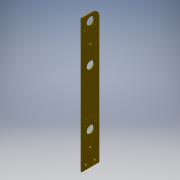
# Autodesk Inventor part: Back Plate
Saved by Autodesk Inventor 2017 (Build 210142000, 142)
## iProperties
Created: 2017-01-13
Part Number: Back Plate
Material: Generic
Document SubType Name: Modeling
Designer: Ben
Density: 1 g/cm^3
Appearance: Gold
Author: Ben
Autodesk Inventor part; units mm, degrees
ref_plane "YZ Plane" through (0, 0, 0) normal (1, 0, 0) x (0, 1, 0)
ref_plane "XZ Plane" through (0, 0, 0) normal (0, 1, 0) x (-1, 0, 0)
ref_plane "XY Plane" through (0, 0, 0) normal (0, 0, 1) x (1, 0, 0)
sketch "Sketch1" plane through (0, 0, 0) normal (1, 0, 0) x (0, 1, 0)
  line L0 (386.842, -25.4) -> (0, -25.4) construction
  circle A0 centre (94.742, -25.4) radius 11.1125
  circle A1 centre (367.792, -25.4) radius 11.1125
  circle A2 centre (256.667, -25.4) radius 11.1125
  circle A3 centre (310.642, -25.4) radius 3.175
  line L1 (0, 0) -> (386.842, 0)
  line L2 (386.842, 0) -> (386.842, -50.8)
  line L3 (386.842, -50.8) -> (0, -50.8)
  line L4 (0, -50.8) -> (0, 0)
  line L5 (78.867, -9.525) -> (110.617, -9.525) construction
  line L6 (110.617, -9.525) -> (110.617, -41.275) construction
  circle A4 centre (110.617, -9.525) radius 1.5875
  circle A5 centre (110.617, -41.275) radius 1.5875
  circle A6 centre (78.867, -9.525) radius 1.5875
  line L7 (351.917, -9.525) -> (351.917, -41.275) construction
  circle A7 centre (351.917, -41.275) radius 1.5875
  circle A8 centre (351.917, -9.525) radius 1.5875
  line L8 (12.7, -50.8) -> (12.7, 0) construction
  circle A9 centre (12.7, -38.1) radius 3.175
  circle A10 centre (12.7, -12.7) radius 3.175
  line L9 (126.492, 0) -> (126.492, -50.8) construction
  line L10 (126.492, -12.7) -> (145.542, -12.7) construction
  circle A11 centre (126.492, -12.7) radius 1.5875
  circle A12 centre (145.542, -12.7) radius 1.5875
  circle A13 centre (126.492, -31.75) radius 1.5875
  circle A14 centre (50.8, -25.4) radius 3.175
  point P0 (351.917, -25.4)
  dimension "d3" = 22.225
  dimension "d4" = 273.05
  dimension "d9" = 161.925
  dimension "d12" = 6.35
  dimension "d13" = 57.15
  dimension "d15" = 50.8
  dimension "d16" = 19.05
  dimension "d17" = 94.742
  dimension "d18" = 3.175
  dimension "d19" = 9.525
  dimension "d20" = 31.75
  dimension "d22" = 15.875
  dimension "d23" = 3.175
  dimension "d24" = 15.875
  dimension "d25" = 31.75
  dimension "d26" = 6.35
  dimension "d27" = 12.7
  dimension "d28" = 25.4
  dimension "d29" = 19.05
  dimension "d30" = 19.05
  dimension "d31" = 6.35
  dimension "d32" = 31.75
  dimension "d33" = 38.1
  constraints: 22 end point, 15 centre point, 14 point on line, 10 equal radius, 7 coincident, 5 perpendicular, 3 horizontal, 3 midpoint, 2 parallel, 1 vertical, 1 other
  measures "d3" diameter of A0
  measures "d4" distance of A0.centre A1.centre
  measures "d9" distance of A0.centre A2.centre
  measures "d12" diameter of A3
  measures "d13" distance of A1.centre A3.centre
  measures "d15" distance of L3.end L1.start
  measures "d16" distance from line of L2 A1.centre
  measures "d17" distance from line of L4 A0.centre
  measures "d18" diameter of A4
  measures "d19" distance between parallel lines of L1 L5
  measures "d20" distance of L5.start L5.end
  measures "d22" horizontal distance of A0.centre L5.start
  measures "d23" diameter of A7
  measures "d24" distance from line of L7 A1.centre
  measures "d25" distance of L7.start L7.end
  measures "d26" diameter of A9
  measures "d27" distance between parallel lines of L4 L8
  measures "d28" distance of A10.centre A9.centre
  measures "d29" distance of L10.start L10.end
  measures "d30" distance of L10.start A13.centre
  measures "d31" distance from line of L0 A13.centre
  measures "d32" distance from line of A0.centre L9
  measures "d33" distance from line of L8 A14.centre
extrude "Extrusion1" add sketch "Sketch1" along normal blind 3.175
fillet "Fillet1" radius 19.05 1 edges at (1.5875, 386.842, -50.8)
equation "\"d30\" = d29"
body "Solid1"
